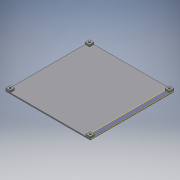
# Autodesk Inventor part: Backplate-housing
Saved by Autodesk Inventor 2016 SP2 (Build 200236200, 236)
## iProperties
Created: 2018-06-21
Part Number: Backplate-housing
Material: Generisch
Document SubType Name: Modeling
Designer: Nils
Density: 1 g/cm^3
Appearance: Vorgabe
Author: Nils
Autodesk Inventor part; units mm, degrees
ref_plane "YZ Plane" through (0, 0, 0) normal (1, 0, 0) x (0, 1, 0)
ref_plane "XZ Plane" through (0, 0, 0) normal (0, 1, 0) x (-1, 0, 0)
ref_plane "XY Plane" through (0, 0, 0) normal (0, 0, 1) x (1, 0, 0)
ref_plane "Arbeitsebene1" through (796.2209, 70.6141, -996.2958) normal (0, 0, -1) x (-1, 0, 0)
sketch "Skizze1" plane through (796.2209, 70.6141, -996.2958) normal (0, 0, -1) x (-1, 0, 0)
  line L0 (-3.9996, -76.75) -> (4.0004, -76.75) construction
  line L1 (-3.9996, 76.75) -> (-3.9996, -76.75) construction
  line L2 (4.0004, 76.75) -> (-3.9996, 76.75) construction
  line L3 (4.0004, 84.25) -> (4.0004, 76.75) construction
  line L4 (-37.8996, 84.25) -> (4.0004, 84.25) construction
  line L5 (-37.8996, 1.75) -> (-37.8996, 84.25) construction
  line L6 (-133.3996, 1.75) -> (-37.8996, 1.75) construction
  line L7 (-133.3996, -84.25) -> (-133.3996, 1.75) construction
  line L8 (4.0004, -84.25) -> (-133.3996, -84.25) construction
  line L9 (4.0004, -76.75) -> (4.0004, -84.25) construction
  line L10 (150.8004, -76.75) -> (142.8004, -76.75) construction
  line L11 (142.8004, -76.75) -> (142.8004, -84.25) construction
  line L12 (142.8004, -84.25) -> (280.2004, -84.25) construction
  line L13 (280.2004, -84.25) -> (280.2004, 1.75) construction
  line L14 (280.2004, 1.75) -> (184.7004, 1.75) construction
  line L15 (184.7004, 1.75) -> (184.7004, 84.25) construction
  line L16 (184.7004, 84.25) -> (142.8004, 84.25) construction
  line L17 (142.8004, 84.25) -> (142.8004, 76.75) construction
  line L18 (142.8004, 76.75) -> (150.8004, 76.75) construction
  line L19 (150.8004, 76.75) -> (150.8004, -76.75) construction
  line L20 (-3.9996, 76.75) -> (150.8004, 76.75)
  line L21 (150.8004, 76.75) -> (150.8004, -76.75)
  line L22 (150.8004, -76.75) -> (-3.9996, -76.75)
  line L23 (-3.9996, -76.75) -> (-3.9996, 76.75)
  point P0 (796.2209, -70.6141)
  constraints: 8 end point, 2 parallel, 1 horizontal, 1 perpendicular
extrude "Extrusion1" add sketch "Skizze1" along normal blind 2
sketch "Skizze2" plane through (796.2209, 70.6141, -996.2958) normal (0, 0, 1) x (1, 0, 0)
  line L0 (-150.8004, 76.75) -> (3.9996, 76.75) projected
  line L1 (3.9996, 76.75) -> (-4.0004, 76.75)
  line L2 (-4.0004, 76.75) -> (-4.0004, 68.75)
  line L3 (-4.0004, 68.75) -> (3.9996, 68.75)
  line L4 (3.9996, 68.75) -> (3.9996, 76.75)
  line L5 (-150.8004, 76.75) -> (-142.8004, 76.75)
  line L6 (-142.8004, 76.75) -> (-142.8004, 68.75)
  line L7 (-142.8004, 68.75) -> (-150.8004, 68.75)
  line L8 (-150.8004, 68.75) -> (-150.8004, 76.75)
  line L9 (3.9996, 76.75) -> (3.9996, -76.75) projected
  line L10 (3.9996, -76.75) -> (-4.0004, -76.75)
  line L11 (-4.0004, -76.75) -> (-4.0004, -68.75)
  line L12 (-4.0004, -68.75) -> (3.9996, -68.75)
  line L13 (3.9996, -68.75) -> (3.9996, -76.75)
  line L14 (3.9996, -76.75) -> (-150.8004, -76.75) projected
  line L15 (-150.8004, -76.75) -> (-142.8004, -76.75)
  line L16 (-142.8004, -76.75) -> (-142.8004, -68.75)
  line L17 (-142.8004, -68.75) -> (-150.8004, -68.75)
  line L18 (-150.8004, -68.75) -> (-150.8004, -76.75)
  point P0 (-796.2209, -70.6141)
  dimension "d2" = 8
  dimension "d3" = 8
  dimension "d4" = 8
  dimension "d5" = 8
  dimension "d6" = 8
  dimension "d7" = 8
  dimension "d8" = 8
  dimension "d9" = 8
  constraints: 32 end point, 8 parallel, 4 horizontal, 4 perpendicular
  measures "d2" distance of L3.end L2.end
  measures "d3" distance of L2.end L1.end
  measures "d4" distance of L6.end L7.end
  measures "d5" distance of L5.end L6.end
  measures "d6" distance of L11.end L12.end
  measures "d7" distance of L10.end L11.end
  measures "d8" distance of L17.end L16.end
  measures "d9" distance of L16.end L15.end
extrude "Extrusion2" add sketch "Skizze2" along normal blind 3.5
sketch "Skizze3" plane through (796.2209, 70.6141, -992.7958) normal (0, 0, 1) x (1, 0, 0)
  circle A0 centre (-146.8004, -72.75) radius 1.75 projected
  circle A1 centre (-0.0004, -72.75) radius 1.75 projected
  circle A2 centre (-0.0004, 72.75) radius 1.75 projected
  circle A3 centre (-146.8004, 72.75) radius 1.75 projected
  point P0 (-796.2209, -70.6141)
extrude "Extrusion3" cut sketch "Skizze3" against normal blind 15.5
sketch "Skizze4" plane through (796.2209, 70.6141, -998.2958) normal (0, 0, -1) x (-1, 0, 0)
  circle A0 centre (0.0004, 72.75) radius 1.75 projected
  circle A1 centre (146.8004, 72.75) radius 1.75 projected
  circle A2 centre (146.8004, -72.75) radius 1.75 projected
  circle A3 centre (0.0004, -72.75) radius 1.75 projected
  circle A4 centre (0.0004, -72.75) radius 1.75 projected
  circle A5 centre (0.0004, -72.75) radius 3
  circle A6 centre (146.8004, -72.75) radius 1.75 projected
  circle A7 centre (146.8004, -72.75) radius 3
  circle A8 centre (0.0004, 72.75) radius 3
  circle A9 centre (146.8004, 72.75) radius 1.75 projected
  circle A10 centre (146.8004, 72.75) radius 3
  point P0 (796.2209, -70.6141)
  dimension "d14" = 6
  dimension "d15" = 6
  dimension "d16" = 6
  dimension "d17" = 6
  constraints: 4 centre point, 4 coincident
  measures "d14" diameter of A5
  measures "d15" diameter of A7
  measures "d16" diameter of A8
  measures "d17" diameter of A10
extrude "Extrusion4" cut sketch "Skizze4" against normal blind 3.4
